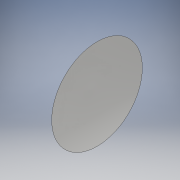
# Autodesk Inventor part: 吸盘
Saved by Autodesk Inventor 2017 (Build 210142000, 142)
## iProperties
Part Number: 吸盘
Material: 常规
Document SubType Name: Modeling
Designer: Administrator
Density: 1 g/cm^3
Appearance: 默认
Author: Administrator
Autodesk Inventor part; units mm, degrees
ref_plane "YZ Plane" through (0, 0, 0) normal (1, 0, 0) x (0, 1, 0)
ref_plane "XZ Plane" through (0, 0, 0) normal (0, 1, 0) x (-1, 0, 0)
ref_plane "XY Plane" through (0, 0, 0) normal (0, 0, 1) x (1, 0, 0)
sketch "草图1" plane through (0, 0, 0) normal (0, 1, 0) x (-1, 0, 0)
  line L0 (0, 0) -> (0, -6)
  line L1 (0, -6) -> (8, -6) construction
  line L2 (0, 0) -> (-2, 0)
  arc A0 (-4, -12.9282) -> (-2, 0) centre (-31.9341, -1.988) ccw
  arc A1 (-4, -12.9282) -> (0, -6) centre (-27.7488, 5.402) ccw
  dimension "d0" = 6
  dimension "d2" = 8
  dimension "d3" = 2
  dimension "d4" = 30
  dimension "d5" = 30
  constraints: 6 end point, 4 point on circle, 2 centre point, 2 horizontal, 1 vertical
  measures "d0" distance of L0.start L0.end
  measures "d2" distance of L0.end A0.start
  measures "d3" distance of L0.start L2.end
  measures "d4" radius of A0
  measures "d5" radius of A1
revolve "旋转1" add sketch "草图1" angle 360 about axis through (0, 0, 0) along (1, 0, 0)
